Autodesk Inventor part; units mm, degrees
(part 3 of 3)
sketch "Sketch8" plane through (0, 0, 0) normal (0, 0, 1) x (1, 0, 0)
  line L0 (6.1983, 26.6612) -> (5.4238, 26.6612) construction
  line L1 (6.1983, 14.8446) -> (6.1983, 26.6612) projected
  line L2 (6.1293, 14.2121) -> (6.1983, 14.8446) construction
  line L3 (5.9709, 13.7973) -> (6.1293, 14.2121) construction
  line L4 (5.9268, 13.7518) -> (5.9709, 13.7973) construction
  line L5 (5.8813, 13.7077) -> (5.9268, 13.7518) construction
  line L6 (5.4417, 13.5533) -> (5.8813, 13.7077) construction
  line L7 (4.7582, 13.4872) -> (5.4417, 13.5533) construction
  line L8 (3.0618, 13.4872) -> (4.7582, 13.4872) projected
  line L9 (3.0618, 11.5607) -> (3.0618, 13.4872) projected
  line L10 (12.9024, 11.5607) -> (3.0618, 11.5607) projected
  line L11 (12.9024, 13.4872) -> (12.9024, 11.5607) projected
  line L12 (11.2267, 13.4872) -> (12.9024, 13.4872) projected
  line L13 (10.5363, 13.5547) -> (11.2267, 13.4872) construction
  line L14 (10.0898, 13.7132) -> (10.5363, 13.5547) construction
  line L15 (10.0444, 13.7587) -> (10.0898, 13.7132) construction
  line L16 (9.9975, 13.8041) -> (10.0444, 13.7587) construction
  line L17 (9.8349, 14.2189) -> (9.9975, 13.8041) construction
  line L18 (9.766, 14.8473) -> (9.8349, 14.2189) construction
  line L19 (9.766, 26.6612) -> (9.766, 14.8473)
  line L20 (10.5736, 26.6612) -> (9.766, 26.6612) construction
  line L21 (11.8854, 26.3526) -> (10.5736, 26.6612) construction
  line L22 (12.9327, 25.6333) -> (11.8854, 26.3526) construction
  line L23 (13.0871, 25.4265) -> (12.9327, 25.6333) construction
  line L24 (13.2414, 25.2212) -> (13.0871, 25.4265) construction
  line L25 (13.7871, 23.828) -> (13.2414, 25.2212) construction
  line L26 (14.0338, 21.9483) -> (13.7871, 23.828) construction
  line L27 (14.0379, 21.4991) -> (14.0338, 21.9483) construction
  line L28 (15.9768, 21.4991) -> (14.0379, 21.4991)
  line L29 (15.9768, 28.5255) -> (15.9768, 21.4991)
  line L30 (0, 28.5255) -> (15.9768, 28.5255) projected
  line L31 (0, 21.4988) -> (0, 28.5255) projected
  line L32 (1.9389, 21.4988) -> (0, 21.4988) projected
  line L33 (1.9444, 21.9535) -> (1.9389, 21.4988) construction
  line L34 (2.198, 23.8497) -> (1.9444, 21.9535) construction
  line L35 (2.7478, 25.2415) -> (2.198, 23.8497) construction
  line L36 (2.9022, 25.4442) -> (2.7478, 25.2415) construction
  line L37 (3.0565, 25.6467) -> (2.9022, 25.4442) construction
  line L38 (4.1051, 26.3565) -> (3.0565, 25.6467) construction
  line L39 (5.4238, 26.6612) -> (4.1051, 26.3565) construction
  line L40 (1.9444, 21.9535) -> (1.9389, 21.4988) construction
  line L41 (2.198, 23.8497) -> (1.9444, 21.9535) construction
  line L42 (2.7478, 25.2415) -> (2.198, 23.8497) construction
  line L43 (4.1051, 26.3565) -> (3.0565, 25.6467) construction
  line L44 (5.4238, 26.6612) -> (4.1051, 26.3565) construction
  line L45 (6.1983, 26.6612) -> (5.4238, 26.6612) construction
  line L46 (11.8854, 26.3526) -> (10.5736, 26.6612) construction
  line L47 (10.5736, 26.6612) -> (9.766, 26.6612) construction
  line L48 (12.9327, 25.6333) -> (11.8854, 26.3526) construction
  line L49 (13.7871, 23.828) -> (13.2414, 25.2212) construction
  line L50 (14.0338, 21.9483) -> (13.7871, 23.828) construction
  line L51 (14.0379, 21.4991) -> (14.0338, 21.9483) construction
  line L52 (6.1293, 14.2121) -> (6.1983, 14.8446) construction
  line L53 (5.9709, 13.7973) -> (6.1293, 14.2121) construction
  line L54 (5.4417, 13.5533) -> (5.8813, 13.7077) construction
  line L55 (4.7582, 13.4872) -> (5.4417, 13.5533) construction
  line L56 (10.5363, 13.5547) -> (11.2267, 13.4872) construction
  line L57 (10.0898, 13.7132) -> (10.5363, 13.5547) construction
  line L58 (10.0444, 13.7587) -> (10.0898, 13.7132) construction
  line L59 (9.9975, 13.8041) -> (10.0444, 13.7587) construction
  line L60 (9.8349, 14.2189) -> (9.9975, 13.8041) construction
  line L61 (9.766, 14.8473) -> (9.8349, 14.2189) construction
  line L62 (1.9389, 21.4988) -> (0, 21.4988)
  line L63 (1.9389, 21.4988) -> (0, 21.4988) projected
  line L64 (0, 21.4988) -> (0, 28.5255)
  line L65 (15.9768, 28.5255) -> (15.9768, 21.4991)
  line L66 (15.9768, 21.4991) -> (14.0379, 21.4991) projected
  line L67 (15.9768, 21.4991) -> (14.0379, 21.4991)
  line L68 (4.7582, 13.4872) -> (3.0618, 13.4872)
  line L69 (12.9024, 11.5607) -> (3.0618, 11.5607) projected
  line L70 (3.0618, 13.4872) -> (3.0618, 11.5607)
  line L71 (3.0618, 11.5607) -> (12.9024, 11.5607)
  line L72 (12.9024, 13.4872) -> (11.2267, 13.4872)
  line L73 (12.9024, 13.4872) -> (12.9024, 11.5607)
  line L74 (9.766, 26.6612) -> (9.766, 14.8473) projected
  line L75 (9.766, 14.8473) -> (9.766, 26.6612)
  line L76 (6.1983, 26.6612) -> (5.811, 26.6612) construction
  line L77 (5.811, 26.6612) -> (5.4238, 26.6612) construction
  line L78 (5.4238, 26.6612) -> (4.1051, 26.3565) construction
  line L79 (4.1051, 26.3565) -> (3.0565, 25.6467) construction
  line L80 (3.0565, 25.6467) -> (2.9022, 25.4442) construction
  line L81 (2.9022, 25.4442) -> (2.7478, 25.2415) construction
  line L82 (2.7478, 25.2415) -> (2.4729, 24.5456) construction
  line L83 (2.4729, 24.5456) -> (2.198, 23.8497) construction
  line L84 (2.198, 23.8497) -> (2.0712, 22.9016) construction
  line L85 (2.0712, 22.9016) -> (1.9444, 21.9535) construction
  line L86 (1.9444, 21.9535) -> (1.9417, 21.7261) construction
  line L87 (1.9417, 21.7261) -> (1.9389, 21.4988) construction
  spline S0 degree 4 poles (6.1983, 26.6612) (5.811, 26.6612) (5.4238, 26.6612) (4.1051, 26.3565) (3.0565, 25.6467) (2.9022, 25.4442) (2.7478, 25.2415) (2.4729, 24.5456) (2.198, 23.8497) (2.0712, 22.9016) (1.9444, 21.9535) (1.9417, 21.7261) (1.9389, 21.4988) knots 1 1 1 1 1 2 3 4 5 6 7 8 9 10 10 10 10 10
  line L88 (6.1983, 26.6612) -> (6.1983, 14.8446)
  line L89 (9.766, 26.6612) -> (10.1698, 26.6612) construction
  line L90 (10.1698, 26.6612) -> (10.5736, 26.6612) construction
  line L91 (10.5736, 26.6612) -> (11.2295, 26.5069) construction
  line L92 (11.2295, 26.5069) -> (11.8854, 26.3526) construction
  line L93 (11.8854, 26.3526) -> (12.4091, 25.9929) construction
  line L94 (12.4091, 25.9929) -> (12.9327, 25.6333) construction
  line L95 (12.9327, 25.6333) -> (13.0871, 25.4265) construction
  line L96 (13.0871, 25.4265) -> (13.2414, 25.2212) construction
  line L97 (13.2414, 25.2212) -> (13.5143, 24.5246) construction
  line L98 (13.5143, 24.5246) -> (13.7871, 23.828) construction
  line L99 (13.7871, 23.828) -> (13.9105, 22.8882) construction
  line L100 (13.9105, 22.8882) -> (14.0338, 21.9483) construction
  line L101 (14.0338, 21.9483) -> (14.0359, 21.7237) construction
  line L102 (14.0359, 21.7237) -> (14.0379, 21.4991) construction
  spline S1 degree 4 poles (9.766, 26.6612) (10.1698, 26.6612) (10.5736, 26.6612) (11.2295, 26.5069) (11.8854, 26.3526) (12.4091, 25.9929) (12.9327, 25.6333) (13.0871, 25.4265) (13.2414, 25.2212) (13.5143, 24.5246) (13.7871, 23.828) (13.9105, 22.8882) (14.0338, 21.9483) (14.0359, 21.7237) (14.0379, 21.4991) knots 1 1 1 1 1 2 3 4 5 6 7 8 9 10 11 12 12 12 12 12
  line L103 (4.7582, 13.4872) -> (5.1, 13.5203) construction
  line L104 (5.1, 13.5203) -> (5.4417, 13.5533) construction
  line L105 (5.4417, 13.5533) -> (5.6615, 13.6305) construction
  line L106 (5.6615, 13.6305) -> (5.8813, 13.7077) construction
  line L107 (5.8813, 13.7077) -> (5.9268, 13.7518) construction
  line L108 (5.9268, 13.7518) -> (5.9709, 13.7973) construction
  line L109 (5.9709, 13.7973) -> (6.0501, 14.0047) construction
  line L110 (6.0501, 14.0047) -> (6.1293, 14.2121) construction
  line L111 (6.1293, 14.2121) -> (6.1638, 14.5283) construction
  line L112 (6.1638, 14.5283) -> (6.1983, 14.8446) construction
  spline S2 degree 4 poles (4.7582, 13.4872) (5.1, 13.5203) (5.4417, 13.5533) (5.6615, 13.6305) (5.8813, 13.7077) (5.9268, 13.7518) (5.9709, 13.7973) (6.0501, 14.0047) (6.1293, 14.2121) (6.1638, 14.5283) (6.1983, 14.8446) knots 1 1 1 1 1 2 3 4 5 6 7 8 8 8 8 8
  line L113 (9.766, 14.8473) -> (9.8004, 14.5331) construction
  spline S3 degree 4 poles (9.766, 14.8473) (9.8004, 14.5331) (9.8349, 14.2189) (9.9162, 14.0115) (9.9975, 13.8041) (10.0444, 13.7587) (10.0898, 13.7132) (10.3131, 13.634) (10.5363, 13.5547) (10.8815, 13.521) (11.2267, 13.4872) knots 1 1 1 1 1 1.286824 1.330759 1.381504 1.474538 1.728419 1.8309 2 2 2 2 2
  line L114 (10.8815, 13.521) -> (11.2267, 13.4872) construction
  line L115 (10.3131, 13.634) -> (10.5363, 13.5547) construction
  line L116 (10.5363, 13.5547) -> (10.8815, 13.521) construction
  line L117 (10.0444, 13.7587) -> (10.0898, 13.7132) construction
  line L118 (10.0898, 13.7132) -> (10.3131, 13.634) construction
  line L119 (9.8004, 14.5331) -> (9.8349, 14.2189) construction
  line L120 (9.8349, 14.2189) -> (9.9162, 14.0115) construction
  line L121 (9.9162, 14.0115) -> (9.9975, 13.8041) construction
  line L122 (9.9975, 13.8041) -> (10.0444, 13.7587) construction
  line L123 (9.766, 26.6612) -> (9.766, 14.8473)
  line L124 (1.9389, 21.4988) -> (0, 21.4988)
  line L125 (0, 21.4988) -> (0, 28.5255)
  line L126 (14.0379, 21.4991) -> (15.9768, 21.4991)
  line L127 (15.9768, 21.4991) -> (15.9768, 28.5255)
  line L128 (4.7582, 13.4872) -> (3.0618, 13.4872)
  line L129 (3.0618, 11.5607) -> (3.0618, 13.4872) projected
  line L130 (3.0618, 13.4872) -> (3.0618, 11.5607)
  line L131 (3.0618, 11.5607) -> (12.9024, 11.5607)
  line L132 (12.9024, 13.4872) -> (12.9024, 11.5607) projected
  line L133 (12.9024, 11.5607) -> (12.9024, 13.4872)
  line L134 (12.9024, 13.4872) -> (11.2267, 13.4872)
  line L135 (9.766, 26.6612) -> (9.766, 14.8473) projected
  line L136 (9.766, 14.8473) -> (9.766, 26.6612)
  line L137 (6.1983, 14.8446) -> (6.1983, 26.6612) projected
  line L138 (6.1983, 26.6612) -> (6.1983, 14.8446)
  line L139 (0, 28.5255) -> (15.9768, 28.5255) projected
  line L140 (15.9768, 28.5255) -> (0, 28.5255)
  line L141 (0, 21.4988) -> (0, 28.5255) projected
  line L142 (0, 28.5255) -> (0, 21.4988)
  line L143 (0, 21.4988) -> (1.9389, 21.4988)
  point P0 (0, 0)
  point P1 (1.9417, 21.7261)
  point P2 (1.9444, 21.9535)
  point P3 (2.0712, 22.9016)
  point P4 (2.4729, 24.5456)
  point P5 (11.2295, 26.5069)
  point P6 (12.4091, 25.9929)
  point P7 (14.0359, 21.7237)
  point P8 (9.8004, 14.5331)
  point P9 (1.9417, 21.7261)
  point P10 (2.0712, 22.9016)
  point P11 (2.4729, 24.5456)
  point P12 (11.2295, 26.5069)
  point P13 (14.0359, 21.7237)
  point P14 (12.4091, 25.9929)
  point P15 (9.8004, 14.5331)
  constraints: 71 coincident, 58 end point, 31 midpoint, 15 point on line, 11 collinear, 5 horizontal, 5 perpendicular, 4 vertical, 17 other
sketch "Sketch9" plane through (0, 0, 0) normal (0, 0, 1) x (1, 0, 0)
  line L0 (0, 28.5255) -> (15.9768, 28.5255)
  line L1 (15.9768, 28.5255) -> (15.9768, 11.5607)
  line L2 (15.9768, 11.5607) -> (0, 11.5607)
  line L3 (0, 11.5607) -> (0, 28.5255)
  line L4 (12.9024, 11.5607) -> (3.0618, 11.5607) projected
  point P0 (0, 0)
  point P1 (15.9768, 21.4991)
  constraints: 8 end point, 2 parallel, 2 point on line, 1 horizontal, 1 perpendicular
extrude "Extrusion6" cut sketch "Sketch9" against normal through all
extrude "Extrusion7" add sketch "Sketch8" against normal blind 25.4
body "Solid1"
